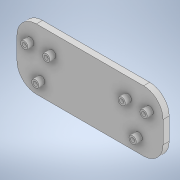
# Autodesk Inventor part: Baseplate
Saved by Autodesk Inventor 2021 (Build 250183000, 183)
## iProperties
Created: 2024-03-24
Part Number: Baseplate
Material: Generic
Document SubType Name: Modeling
Designer: Lukas
Density: 1 g/cm^3
Appearance: Default
Author: Lukas
Autodesk Inventor part; units mm, degrees
ref_plane "YZ Plane" through (0, 0, 0) normal (1, 0, 0) x (0, 1, 0)
ref_plane "XZ Plane" through (0, 0, 0) normal (0, 1, 0) x (-1, 0, 0)
ref_plane "XY Plane" through (0, 0, 0) normal (0, 0, 1) x (1, 0, 0)
sketch "Sketch1" plane through (0, 0, 0) normal (0, 0, 1) x (1, 0, 0)
  circle A0 centre (-49, 10) radius 1.65
  circle A1 centre (-31, 10) radius 1.65
  circle A2 centre (-49, 10) radius 3
  circle A3 centre (-31, 10) radius 3
  line L0 (-60, 25) -> (60, 25)
  line L1 (60, 25) -> (60, -25)
  line L2 (60, -25) -> (-60, -25)
  line L3 (-60, -25) -> (-60, 25)
  circle A4 centre (31, 10) radius 1.65
  circle A5 centre (31, 10) radius 3
  circle A6 centre (49, 10) radius 1.65
  circle A7 centre (49, 10) radius 3
  circle A8 centre (40, -13) radius 1.65
  circle A9 centre (40, -13) radius 3
  circle A10 centre (-40, -13) radius 1.65
  circle A11 centre (-40, -13) radius 3
  point P0 (0, 0)
  point P1 (0, 25)
  point P2 (-60, 0)
  dimension "d2" = 10
  dimension "d5" = 3.3
  dimension "d6" = 6
  dimension "d44" = 50
  dimension "d45" = 120
  dimension "d46" = 18
  dimension "d50" = 18
  dimension "d51" = 9
  dimension "d52" = 20
  dimension "d53" = 9
  dimension "d54" = 13
  dimension "d55" = 20
  constraints: 12 centre point, 10 equal radius, 8 end point, 6 coincident, 5 horizontal alignment, 2 midpoint, 2 parallel, 1 horizontal, 1 perpendicular, 1 vertical alignment
  measures "d2" vertical distance of A1.centre point (0, 0)
  measures "d5" diameter of A0
  measures "d6" diameter of A2
  measures "d44" distance of L2.end L0.start
  measures "d45" distance of L0.start L0.end
  measures "d46" distance of A1.centre A0.centre
  measures "d50" distance of A6.centre A4.centre
  measures "d51" horizontal distance of A6.centre A8.centre
  measures "d52" distance from line of L1 A9.centre
  measures "d53" horizontal distance of A10.centre A0.centre
  measures "d54" vertical distance of point (0, 0) A10.centre
  measures "d55" distance from line of L3 A10.centre
extrude "Extrusion1" add sketch "Sketch1" along normal blind 5 contours A2 | A3 | L0 L1 L2 L3 | A5 | A7 | A9 | A11
extrude "Extrusion2" add sketch "Sketch1" along normal blind 10 contours A2 | A3 | A5 | A7 | A9 | A11
extrude "Extrusion7" cut sketch "Sketch1" along normal blind 3 contours A0 | A1 | A2 | A3 | A4 | A5 | A6 | A7 | A8 | A9 | A10 | A11
fillet "Fillet1" radius 16 4 edges at (-60, 25, 2.5) (-60, -25, 2.5) (60, 25, 2.5) (60, -25, 2.5)
equation "\"d50\" = d46"
equation "\"d51\" = d53"
equation "\"d52\" = d49"
equation "\"d53\" = 0.5 * d46"
equation "\"d47\" = 0.5 * d46"
equation "\"d49\" = 20"
body "Solid1"
